Autodesk Inventor part; units mm, degrees
(part 2 of 3)
sketch "Sketch15" plane through (0, 0, 304.8) normal (0, 0, 1) x (1, 0, 0)
  arc A0 (-46.3112, 3289.8328) -> (-107.6796, 3264.8246) centre (12.3811, 3058.0053) ccw
  arc A1 (-107.6796, 3264.8246) -> (-166.2681, 3221.918) centre (64.3962, 2968.4026) ccw
  arc A2 (-166.2681, 3221.918) -> (-212.0324, 3170.0211) centre (46.0659, 2988.5486) ccw
  arc A3 (-212.0324, 3170.0211) -> (-234.7582, 3118.3718) centre (-94.8804, 3087.6496) ccw
  arc A4 (-240.3697, 3101.0693) -> (-234.7582, 3118.3718) centre (-326.0966, 3138.4331) ccw
  arc A5 (-248.2053, 3093.022) -> (-240.3697, 3101.0693) centre (-254.9435, 3107.4212) ccw
  arc A6 (-262.3292, 3089.5785) -> (-248.2053, 3093.022) centre (-263.8246, 3126.4001) ccw
  arc A7 (-297.9256, 3088.8125) -> (-262.3292, 3089.5785) centre (-300.2034, 4022.1257) ccw
  arc A8 (-297.9256, 3088.8125) -> (-398.3817, 3086.3759) centre (-292.3004, 784.8853) ccw
  arc A9 (-398.3817, 3086.3759) -> (-582.9034, 3077.1219) centre (652.3851, -19709.8746) ccw
  arc A10 (-582.9034, 3077.1219) -> (-779.8872, 3065.5252) centre (566.6285, -18127.8528) ccw
  arc A11 (-779.8872, 3065.5252) -> (-944.631, 3053.7542) centre (-115.3773, -7393.4842) ccw
  arc A12 (-944.631, 3053.7542) -> (-1250.7142, 3024.3128) centre (-215.4099, -6133.2828) ccw
  arc A13 (-1250.7142, 3024.3128) -> (-1574.5871, 2983.1171) centre (64.6721, -8610.7314) ccw
  arc A14 (-1574.5871, 2983.1171) -> (-1876.7817, 2935.965) centre (-80.0841, -7586.984) ccw
  arc A15 (-1876.7817, 2935.965) -> (-2112.8509, 2888.5788) centre (-1177.7038, -1158.4352) ccw
  arc A16 (-2163.2488, 2877.2292) -> (-2112.8509, 2888.5788) centre (-3155.0339, 7398.8142) ccw
  arc A17 (-2208.5733, 2867.6541) -> (-2163.2488, 2877.2292) centre (-2805.2472, 5804.1243) ccw
  arc A18 (-2246.7459, 2860.0907) -> (-2208.5733, 2867.6541) centre (-3005.4604, 6789.4539) ccw
  arc A19 (-2258.6611, 2858.9509) -> (-2246.7459, 2860.0907) centre (-2258.6611, 2921.7997) ccw
  arc A20 (-2266.3764, 2860.7683) -> (-2258.6611, 2858.9509) centre (-2258.6611, 2876.2361) ccw
  arc A21 (-2275.0416, 2866.3453) -> (-2266.3764, 2860.7683) centre (-2245.2702, 2903.0826) ccw
  arc A22 (-2283.2654, 2874.4944) -> (-2275.0416, 2866.3453) centre (-2238.4614, 2911.4846) ccw
  arc A23 (-2289.7233, 2884.1233) -> (-2283.2654, 2874.4944) centre (-2238.2095, 2911.6926) ccw
  arc A24 (-2289.7233, 2884.1233) -> (-2321.8745, 2924.2434) centre (-2413.4792, 2817.891) ccw
  arc A25 (-2321.8745, 2924.2434) -> (-2371.8848, 2958.161) centre (-2493.5929, 2724.8793) ccw
  arc A26 (-2371.8848, 2958.161) -> (-2431.0862, 2981.1586) centre (-2505.2634, 2702.5101) ccw
  arc A27 (-2431.0862, 2981.1586) -> (-2490.6497, 2988.9509) centre (-2490.6498, 2757.4058) ccw
  arc A28 (-2490.6497, 2988.9509) -> (-2542.4535, 2985.3232) centre (-2490.6494, 2617.2557) ccw
  arc A29 (-2542.4535, 2985.3232) -> (-2586.7085, 2974.3691) centre (-2511.4982, 2765.3889) ccw
  arc A30 (-2586.7085, 2974.3691) -> (-2626.6985, 2954.9638) centre (-2515.7885, 2777.3109) ccw
  arc A31 (-2626.6985, 2954.9638) -> (-2665.6409, 2925.9729) centre (-2469.4507, 2703.0889) ccw
  arc A32 (-2665.6409, 2925.9729) -> (-2702.3557, 2887.9704) centre (-2449.4743, 2680.3944) ccw
  arc A33 (-2702.3557, 2887.9704) -> (-2729.3602, 2847.2341) centre (-2516.7134, 2735.5871) ccw
  arc A34 (-2729.3602, 2847.2341) -> (-2747.2851, 2802.3677) centre (-2522.1108, 2738.4208) ccw
  arc A35 (-2747.2851, 2802.3677) -> (-2756.9469, 2752.0682) centre (-2463.5322, 2721.785) ccw
  line L0 (-2756.9469, 2752.0682) -> (-2762.5543, 2697.7376)
  line L1 (-2762.5543, 2697.7376) -> (-2857.3018, 2653.4618)
  arc A36 (-2857.3018, 2653.4618) -> (-2992.0543, 2581.5731) centre (-2246.1893, 1345.7176) ccw
  arc A37 (-2992.0543, 2581.5731) -> (-3103.2533, 2502.66) centre (-2516.6696, 1793.8896) ccw
  arc A38 (-3103.2533, 2502.66) -> (-3188.8522, 2418.6621) centre (-2650.8401, 1956.0099) ccw
  arc A39 (-3188.8522, 2418.6621) -> (-3246.4159, 2331.4275) centre (-2875.8904, 2149.5375) ccw
  line L2 (-3246.4159, 2331.4275) -> (-3274.631, 2273.9509)
  line L3 (-3274.631, 2273.9509) -> (-3274.631, 1968.9509)
  arc A40 (-3274.631, 1968.9509) -> (-3273.1115, 1744.3083) centre (13331.6928, 1968.9509) ccw
  arc A41 (-3273.1115, 1744.3083) -> (-3264.9339, 1658.0418) centre (-2737.5712, 1751.554) ccw
  arc A42 (-3264.9339, 1658.0418) -> (-3243.4484, 1598.0315) centre (-3077.6061, 1691.2592) ccw
  arc A43 (-3243.4484, 1598.0315) -> (-3196.1509, 1526.3644) centre (-2717.5396, 1893.6705) ccw
  line L4 (-3196.1509, 1526.3644) -> (-3159.631, 1478.7779)
  line L5 (-3159.631, 1478.7779) -> (-3159.631, 232.7481)
  line L6 (-3159.631, 232.7481) -> (-3159.631, -1013.2817)
  line L7 (-3159.631, -1013.2817) -> (-3194.6687, -1106.8292)
  arc A44 (-3194.6687, -1106.8292) -> (-3235.7053, -1228.3112) centre (-1352.9181, -1796.6438) ccw
  arc A45 (-3235.7053, -1228.3112) -> (-3254.4602, -1317.8486) centre (-2729.893, -1380.9943) ccw
  arc A46 (-3254.4602, -1317.8486) -> (-3262.6146, -1433.5138) centre (-2089.2145, -1458.1182) ccw
  arc A47 (-3262.6146, -1433.5138) -> (-3266.9659, -1707.4159) centre (23693.9, -1998.7406) ccw
  arc A48 (-3266.9659, -1707.4159) -> (-3268.5559, -1915.4498) centre (29628.1072, -2062.8585) ccw
  arc A49 (-3268.5559, -1915.4498) -> (-3267.3161, -2035.0331) centre (758.7581, -1933.4937) ccw
  arc A50 (-3267.3161, -2035.0331) -> (-3263.1758, -2116.2659) centre (-1685.718, -1995.1434) ccw
  arc A51 (-3263.1758, -2116.2659) -> (-3254.9956, -2182.0248) centre (-2561.9283, -2062.4215) ccw
  arc A52 (-3254.9956, -2182.0248) -> (-3203.1859, -2382.1563) centre (-2017.8834, -1968.535) ccw
  arc A53 (-3203.1859, -2382.1563) -> (-3118.1576, -2576.8834) centre (-1881.2535, -1920.8569) ccw
  arc A54 (-3118.1576, -2576.8834) -> (-3000.6889, -2764.0458) centre (-1776.8359, -1865.4747) ccw
  arc A55 (-3000.6889, -2764.0458) -> (-2852.131, -2941.6043) centre (-1527.6023, -1682.4847) ccw
  line L8 (-2852.131, -2941.6043) -> (-2759.631, -3038.9096)
  line L9 (-2759.631, -3038.9096) -> (-2759.631, -3148.0159)
  arc A56 (-2759.631, -3148.0159) -> (-2758.7481, -3211.3797) centre (-485.5874, -3148.0178) ccw
  arc A57 (-2758.7481, -3211.3797) -> (-2755.3551, -3247.6045) centre (-2481.0428, -3203.6394) ccw
  arc A58 (-2755.3551, -3247.6045) -> (-2747.9013, -3276.2194) centre (-2602.9015, -3223.1703) ccw
  arc A59 (-2747.9013, -3276.2194) -> (-2733.8535, -3308.8509) centre (-2448.718, -3166.7618) ccw
  arc A60 (-2733.8535, -3308.8509) -> (-2656.0182, -3402.6512) centre (-2494.9406, -3189.7953) ccw
  arc A61 (-2656.0182, -3402.6512) -> (-2544.9951, -3451.4517) centre (-2497.9927, -3193.8282) ccw
  arc A62 (-2544.9951, -3451.4517) -> (-2424.0985, -3444.948) centre (-2498.1767, -3194.8371) ccw
  arc A63 (-2424.0985, -3444.948) -> (-2318.7115, -3384.5922) centre (-2499.0501, -3191.8895) ccw
  line L10 (-2318.7115, -3384.5922) -> (-2292.792, -3360.3356)
  line L11 (-2292.792, -3360.3356) -> (-2228.7115, -3394.9426)
  arc A64 (-2228.7115, -3394.9426) -> (-2141.5432, -3438.4245) centre (-1515.7339, -2074.7467) ccw
  arc A65 (-2141.5432, -3438.4245) -> (-2023.9363, -3490.359) centre (-279.2994, 619.5343) ccw
  arc A66 (-2023.9363, -3490.359) -> (-1897.8735, -3541.7652) centre (-157.0169, 907.5921) ccw
  arc A67 (-1897.8735, -3541.7652) -> (-1782.4495, -3584.3792) centre (-735.1306, -569.9907) ccw
  arc A68 (-1782.4495, -3584.3792) -> (-1501.5658, -3670.687) centre (-452.9966, 242.0338) ccw
  arc A69 (-1501.5658, -3670.687) -> (-1204.3636, -3740.1039) centre (-281.5333, 881.8376) ccw
  arc A70 (-1204.3636, -3740.1039) -> (-893.0578, -3792.182) centre (-217.5273, 1202.3994) ccw
  arc A71 (-893.0578, -3792.182) -> (-569.8728, -3826.4861) centre (-133.7905, 1821.478) ccw
  arc A72 (-319.0343, -3846.0577) -> (-569.8728, -3826.4861) centre (-12555.6397, -159058.0844) ccw
  arc A73 (-268.9912, -3851.9794) -> (-319.0343, -3846.0577) centre (-369.6818, -4488.4814) ccw
  arc A74 (-247.4204, -3861.4112) -> (-268.9912, -3851.9794) centre (-276.2744, -3898.0189) ccw
  arc A75 (-236.4852, -3879.2256) -> (-247.4204, -3861.4112) centre (-266.1467, -3885.1696) ccw
  arc A76 (-236.4852, -3879.2256) -> (-224.011, -3912.1165) centre (-131.3204, -3858.1516) ccw
  arc A77 (-224.011, -3912.1165) -> (-197.1839, -3951.7522) centre (81.3306, -3734.3454) ccw
  arc A78 (-197.1839, -3951.7522) -> (-163.6615, -3989.2021) centre (97.3029, -3721.8771) ccw
  arc A79 (-163.6615, -3989.2021) -> (-129.7306, -4015.9862) centre (-19.7812, -3841.8149) ccw
  arc A80 (-129.7306, -4015.9862) -> (-22.8543, -4054.6276) centre (11.689, -3791.9632) ccw
  arc A81 (-22.8543, -4054.6276) -> (89.6103, -4044.5426) centre (10.8492, -3798.3496) ccw
  arc A82 (89.6103, -4044.5426) -> (188.2078, -3987.1875) centre (8.9809, -3792.5094) ccw
  arc A83 (188.2078, -3987.1875) -> (255.8747, -3892.625) centre (-4.6846, -3777.6663) ccw
  arc A84 (274.2339, -3865.5547) -> (255.8747, -3892.625) centre (339.2509, -3929.4105) ccw
  arc A85 (298.361, -3852.3578) -> (274.2339, -3865.5547) centre (308.0992, -3898.8151) ccw
  arc A86 (346.2469, -3845.5982) -> (298.361, -3852.3578) centre (373.1383, -4209.0913) ccw
  arc A87 (550.369, -3830.8943) -> (346.2469, -3845.5982) centre (4245.7889, -56555.6607) ccw
  arc A88 (550.369, -3830.8943) -> (1011.9622, -3779.143) centre (160.6183, 1729.9233) ccw
  arc A89 (1011.9622, -3779.143) -> (1450.7614, -3690.264) centre (276.8483, 977.7708) ccw
  arc A90 (1450.7614, -3690.264) -> (1856.9933, -3566.6691) centre (393.1521, 515.2843) ccw
  arc A91 (1856.9933, -3566.6691) -> (2220.8715, -3410.7969) centre (749.9478, -479.643) ccw
  line L12 (2220.8715, -3410.7969) -> (2317.8832, -3362.1141)
  line L13 (2317.8832, -3362.1141) -> (2340.395, -3386.0768)
  arc A92 (2340.395, -3386.0768) -> (2398.6598, -3427.8945) centre (2475.8998, -3258.7765) ccw
  arc A93 (2398.6598, -3427.8945) -> (2476.161, -3451.1721) centre (2522.0514, -3157.7269) ccw
  arc A94 (2476.161, -3451.1721) -> (2558.9087, -3452.9409) centre (2524.1075, -3144.5807) ccw
  arc A95 (2558.9087, -3452.9409) -> (2632.5758, -3431.7696) centre (2533.124, -3224.4709) ccw
  arc A96 (2632.5758, -3431.7696) -> (2672.6678, -3407.2012) centre (2533.1516, -3224.5277) ccw
  arc A97 (2672.6678, -3407.2012) -> (2711.9464, -3372.3297) centre (2456.4615, -3124.1138) ccw
  arc A98 (2711.9464, -3372.3297) -> (2745.4004, -3332.3528) centre (2459.6723, -3127.2323) ccw
  arc A99 (2745.4004, -3332.3528) -> (2767.9369, -3292.4447) centre (2573.5904, -3209.0123) ccw
  arc A100 (2767.9369, -3292.4447) -> (2774.851, -3270.202) centre (2664.9715, -3248.2421) ccw
  arc A101 (2774.851, -3270.202) -> (2780.6818, -3235.3215) centre (2226.4162, -3160.5947) ccw
  arc A102 (2780.6818, -3235.3215) -> (2785.2966, -3191.8844) centre (2012.2156, -3131.7156) ccw
  arc A103 (2785.2966, -3191.8844) -> (2788.3077, -3141.3505) centre (1395.4115, -3083.711) ccw
  line L14 (2788.3077, -3141.3505) -> (2793.054, -3026.652)
  line L15 (2793.054, -3026.652) -> (2881.9987, -2931.3505)
  arc A104 (2881.9987, -2931.3505) -> (3026.1461, -2756.7165) centre (1521.0591, -1661.188) ccw
  arc A105 (3026.1461, -2756.7165) -> (3141.0373, -2573.2817) centre (1768.6588, -1841.4137) ccw
  arc A106 (3141.0373, -2573.2817) -> (3224.9271, -2383.8991) centre (1886.8926, -1904.4681) ccw
  arc A107 (3224.9271, -2383.8991) -> (3276.549, -2191.4998) centre (2079.1422, -1973.3533) ccw
  arc A108 (3276.549, -2191.4998) -> (3290.3678, -2067.3509) centre (2389.8588, -2029.96) ccw
  arc A109 (3290.3678, -2067.3509) -> (3297.8944, -1821.3895) centre (-7979.8895, -1599.3782) ccw
  arc A110 (3297.8944, -1821.3895) -> (3299.7736, -1574.0698) centre (-6932.4546, -1619.9901) ccw
  arc A111 (3299.7736, -1574.0698) -> (3291.643, -1424.7762) centre (1801.6108, -1580.7922) ccw
  arc A112 (3291.643, -1424.7762) -> (3279.1795, -1335.9693) centre (2021.1062, -1557.8098) ccw
  arc A113 (3279.1795, -1335.9693) -> (3260.4248, -1247.3936) centre (1972.1003, -1566.4515) ccw
  arc A114 (3260.4248, -1247.3936) -> (3235.7287, -1160.5183) centre (1978.3425, -1564.905) ccw
  arc A115 (3235.7287, -1160.5183) -> (3205.467, -1076.8057) centre (2049.2486, -1542.0999) ccw
  line L16 (3205.467, -1076.8057) -> (3177.6016, -1007.5624)
  line L17 (3177.6016, -1007.5624) -> (3183.3958, 240.5471)
  line L18 (3183.3958, 240.5471) -> (3189.19, 1488.6566)
  line L19 (3189.19, 1488.6566) -> (3220.1008, 1527.121)
  arc A116 (3220.1008, 1527.121) -> (3233.5209, 1545.7307) centre (3048.6242, 1664.9232) ccw
  arc A117 (3233.5209, 1545.7307) -> (3248.3718, 1570.2027) centre (2790.547, 1831.2912) ccw
  arc A118 (3248.3718, 1570.2027) -> (3262.2919, 1596.2159) centre (2772.5487, 1841.5547) ccw
  arc A119 (3262.2919, 1596.2159) -> (3272.9357, 1619.7682) centre (2973.0626, 1741.1062) ccw
  arc A120 (3272.9357, 1619.7682) -> (3285.3139, 1660.1743) centre (3048.0912, 1710.7471) ccw
  arc A121 (3285.3139, 1660.1743) -> (3292.0528, 1706.3262) centre (2934.4481, 1734.9744) ccw
  arc A122 (3292.0528, 1706.3262) -> (3295.7316, 1779.1786) centre (2058.9549, 1805.1132) ccw
  arc A123 (3295.7316, 1779.1786) -> (3298.506, 1938.9509) centre (-18868.7762, 2243.9706) ccw
  arc A124 (3298.506, 1938.9509) -> (3299.3295, 2124.9239) centre (-6667.2613, 2076.0683) ccw
  arc A125 (3299.3295, 2124.9239) -> (3293.7335, 2225.5886) centre (2303.2827, 2120.0404) ccw
  arc A126 (3293.7335, 2225.5886) -> (3279.7247, 2296.0862) centre (2896.0955, 2183.2137) ccw
  arc A127 (3279.7247, 2296.0862) -> (3253.3427, 2362.7578) centre (2899.7829, 2184.2986) ccw
  arc A128 (3253.3427, 2362.7578) -> (3201.8504, 2436.6131) centre (2968.2007, 2218.8331) ccw
  arc A129 (3201.8504, 2436.6131) -> (3120.5863, 2511.187) centre (2684.435, 1954.3428) ccw
  arc A130 (3120.5863, 2511.187) -> (3012.8103, 2584.6184) centre (2514.227, 1737.0353) ccw
  arc A131 (3012.8103, 2584.6184) -> (2880.2295, 2655.0014) centre (2141.5699, 1103.522) ccw
  line L20 (2880.2295, 2655.0014) -> (2780.369, 2702.545)
  line L21 (2780.369, 2702.545) -> (2780.1493, 2748.2479)
  arc A132 (2780.1493, 2748.2479) -> (2775.0931, 2791.6815) centre (2582.9337, 2747.3004) ccw
  arc A133 (2775.0931, 2791.6815) -> (2760.5416, 2834.592) centre (2553.9, 2740.5949) ccw
  arc A134 (2760.5416, 2834.592) -> (2737.1518, 2875.1119) centre (2539.7972, 2734.1798) ccw
  arc A135 (2737.1518, 2875.1119) -> (2705.9098, 2911.4545) centre (2520.0411, 2720.0719) ccw
  arc A136 (2705.9098, 2911.4545) -> (2667.4339, 2943.5189) centre (2476.1982, 2674.9279) ccw
  arc A137 (2667.4339, 2943.5189) -> (2628.0644, 2965.8563) centre (2539.3212, 2763.5843) ccw
  arc A138 (2628.0644, 2965.8563) -> (2584.5734, 2979.8878) centre (2537.3397, 2759.0682) ccw
  arc A139 (2584.5734, 2979.8878) -> (2533.6971, 2987.0098) centre (2509.5141, 2628.9801) ccw
  arc A140 (2533.6971, 2987.0098) -> (2468.8699, 2982.8618) centre (2516.9837, 2739.5663) ccw
  arc A141 (2468.8699, 2982.8618) -> (2406.3831, 2962.0597) centre (2519.6551, 2726.0573) ccw
  arc A142 (2406.3831, 2962.0597) -> (2350.9834, 2926.2821) centre (2519.9793, 2725.382) ccw
  arc A143 (2350.9834, 2926.2821) -> (2306.9568, 2878.1833) centre (2512.6195, 2734.1315) ccw
  line L22 (2306.9568, 2878.1833) -> (2291.8513, 2856.6172)
  line L23 (2291.8513, 2856.6172) -> (2153.3688, 2887.2409)
  arc A144 (2153.3688, 2887.2409) -> (1789.0499, 2956.0222) centre (863.5291, -2945.494) ccw
  arc A145 (1789.0499, 2956.0222) -> (1366.7853, 3013.4039) centre (178.3761, -7314.3462) ccw
  arc A146 (1366.7853, 3013.4039) -> (909.4742, 3057.1147) centre (4.1851, -8828.2906) ccw
  arc A147 (909.4742, 3057.1147) -> (438.4615, 3084.5728) centre (-97.6129, -10164.7522) ccw
  line L24 (438.4615, 3084.5728) -> (271.5539, 3091.326)
  line L25 (271.5539, 3091.326) -> (245.4506, 3144.6794)
  arc A148 (245.4506, 3144.6794) -> (194.1184, 3215.755) centre (13.3359, 3031.1162) ccw
  arc A149 (194.1184, 3215.755) -> (120.5657, 3268.0706) centre (-8.3291, 3008.9888) ccw
  arc A150 (120.5657, 3268.0706) -> (36.2378, 3294.2646) centre (-2.5085, 3020.6882) ccw
  arc A151 (36.2378, 3294.2646) -> (-46.3112, 3289.8328) centre (6.2222, 3082.3333) ccw
  arc A152 (89.3189, 3150.4436) -> (63.1902, 3165.2397) centre (10.7465, 3042.1598) ccw
  arc A153 (116.9335, 3127.4656) -> (89.3189, 3150.4436) centre (-69.9138, 2930.998) ccw
  arc A154 (138.8775, 3104.1724) -> (116.9335, 3127.4656) centre (-83.9919, 2916.1953) ccw
  arc A155 (138.4328, 3093.6815) -> (138.8775, 3104.1724) centre (132.9453, 3099.1689) ccw
  arc A156 (133.5538, 3091.581) -> (138.4328, 3093.6815) centre (133.3552, 3098.7591) ccw
  arc A157 (97.1027, 3090.7293) -> (133.5538, 3091.581) centre (16.2051, 7333.5774) ccw
  arc A158 (54.6327, 3090.4516) -> (97.1027, 3090.7293) centre (64.784, 4785.7998) ccw
  arc A159 (5.2451, 3091.142) -> (54.6327, 3090.4516) centre (73.1416, 6181.3364) ccw
  line L26 (5.2451, 3091.142) -> (-122.5944, 3093.9509)
  line L27 (-122.5944, 3093.9509) -> (-95.2836, 3126.3799)
  arc A160 (-61.8221, 3155.7464) -> (-95.2836, 3126.3799) centre (18.2392, 3030.774) ccw
  arc A161 (-22.1385, 3172.7641) -> (-61.8221, 3155.7464) centre (9.2314, 3044.835) ccw
  arc A162 (20.6657, 3175.9635) -> (-22.1385, 3172.7641) centre (8.8195, 3046.5143) ccw
  arc A163 (63.1902, 3165.2397) -> (20.6657, 3175.9635) centre (7.7851, 3035.21) ccw
  arc A164 (1482.1495, 2879.5394) -> (835.369, 2944.786) centre (-222.8049, -10783.103) ccw
  arc A165 (2033.8348, 2789.8546) -> (1482.1495, 2879.5394) centre (546.8422, -4615.54) ccw
  arc A166 (2488.7788, 2677.7909) -> (2033.8348, 2789.8546) centre (969.6677, -2509.8371) ccw
  arc A167 (2835.369, 2543.1909) -> (2488.7788, 2677.7909) centre (1877.3908, 589.9613) ccw
  arc A168 (2972.4358, 2468.9016) -> (2835.369, 2543.1909) centre (1991.5457, 822.7108) ccw
  arc A169 (3070.8462, 2398.2555) -> (2972.4358, 2468.9016) centre (2608.3198, 1857.8197) ccw
  arc A170 (3136.2171, 2328.1438) -> (3070.8462, 2398.2555) centre (2793.243, 2073.8919) ccw
  arc A171 (3171.2321, 2255.7454) -> (3136.2171, 2328.1438) centre (2962.8708, 2199.6394) ccw
  arc A172 (3167.3401, 2165.8281) -> (3171.2321, 2255.7454) centre (3027.1211, 2216.9403) ccw
  arc A173 (3112.4013, 2072.38) -> (3167.3401, 2165.8281) centre (2885.8896, 2268.4214) ccw
  arc A174 (3006.3187, 1977.6944) -> (3112.4013, 2072.38) centre (2693.5168, 2434.916) ccw
  arc A175 (2849.8778, 1884.4435) -> (3006.3187, 1977.6944) centre (2182.6997, 3181.5742) ccw
  line L28 (2849.8778, 1884.4435) -> (2744.3866, 1830.1842)
  line L29 (2744.3866, 1830.1842) -> (2718.8658, 1862.1684)
  arc A176 (2718.8658, 1862.1684) -> (2705.319, 1876.4972) centre (2626.883, 1788.7735) ccw
  arc A177 (2705.319, 1876.4972) -> (2685.042, 1893.3565) centre (2460.6821, 1602.8924) ccw
  arc A178 (2685.042, 1893.3565) -> (2662.0222, 1909.8756) centre (2439.3453, 1575.269) ccw
  arc A179 (2662.0222, 1909.8756) -> (2639.5587, 1923.4268) centre (2498.2071, 1663.7176) ccw
  arc A180 (2639.5587, 1923.4268) -> (2522.8271, 1952.9332) centre (2523.618, 1710.4053) ccw
  arc A181 (2522.8271, 1952.9332) -> (2402.6794, 1924.0014) centre (2523.6996, 1685.3691) ccw
  arc A182 (2402.6794, 1924.0014) -> (2308.0062, 1844.0185) centre (2524.5087, 1683.7737) ccw
  arc A183 (2308.0062, 1844.0185) -> (2261.9871, 1731.9451) centre (2506.7243, 1696.9371) ccw
  line L30 (2261.9871, 1731.9451) -> (2255.1849, 1684.392)
  line L31 (2255.1849, 1684.392) -> (2180.277, 1666.9309)
  arc A184 (2080.1328, 1646.3683) -> (2180.277, 1666.9309) centre (1742.2701, 3545.9722) ccw
  arc A185 (1895.2662, 1614.4296) -> (2080.1328, 1646.3683) centre (-1243.6324, 20333.9108) ccw
  arc A186 (1705.5784, 1583.7089) -> (1895.2662, 1614.4296) centre (-954.2792, 18608.2412) ccw
  arc A187 (1570.369, 1564.661) -> (1705.5784, 1583.7089) centre (1004.2625, 6072.516) ccw
  arc A188 (1325.9578, 1537.6216) -> (1570.369, 1564.661) centre (531.3741, 9838.0633) ccw
  arc A189 (1053.4411, 1514.482) -> (1325.9578, 1537.6216) centre (111.4621, 14224.5078) ccw
  arc A190 (765.7527, 1496.1277) -> (1053.4411, 1514.482) centre (15.6875, 15516.6442) ccw
  arc A191 (475.369, 1483.5075) -> (765.7527, 1496.1277) centre (-9.5547, 15988.3407) ccw
  line L32 (475.369, 1483.5075) -> (275.369, 1476.8212)
  line L33 (275.369, 1476.8212) -> (254.0585, 1520.7051)
  arc A192 (254.0585, 1520.7051) -> (210.3619, 1589.1404) centre (-60.9732, 1367.7223) ccw
  arc A193 (210.3619, 1589.1404) -> (155.3377, 1638.8441) centre (20.3039, 1434.0467) ccw
  arc A194 (155.3377, 1638.8441) -> (89.5075, 1668.7278) centre (27.9039, 1445.5724) ccw
  arc A195 (89.5075, 1668.7278) -> (14.0565, 1678.9509) centre (14.0566, 1395.4107) ccw
  arc A196 (14.0565, 1678.9509) -> (-11.8929, 1678.1751) centre (14.0563, 1244.6069) ccw
  arc A197 (-11.8929, 1678.1751) -> (-38.2726, 1675.8493) centre (16.1999, 1208.7817) ccw
  arc A198 (-38.2726, 1675.8493) -> (-61.5157, 1672.4671) centre (9.6394, 1265.031) ccw
  arc A199 (-61.5157, 1672.4671) -> (-76.48, 1668.3921) centre (-47.1455, 1590.1833) ccw
  arc A200 (-76.48, 1668.3921) -> (-128.8275, 1641.0381) centre (8.2697, 1442.4402) ccw
  arc A201 (-128.8275, 1641.0381) -> (-177.1616, 1600.019) centre (52.4265, 1378.4747) ccw
  arc A202 (-177.1616, 1600.019) -> (-214.9194, 1551.8877) centre (38.2305, 1392.1732) ccw
  arc A203 (-214.9194, 1551.8877) -> (-235.6528, 1503.44) centre (-73.7028, 1462.793) ccw
  line L34 (-235.6528, 1503.44) -> (-242.4619, 1476.3107)
  line L35 (-242.4619, 1476.3107) -> (-443.5464, 1482.9751)
  arc A204 (-781.6776, 1498.1041) -> (-443.5464, 1482.9751) centre (40.3784, 16084.7975) ccw
  arc A205 (-1113.5104, 1520.8708) -> (-781.6776, 1498.1041) centre (-15.0259, 15102.0022) ccw
  arc A206 (-1424.5661, 1550.0611) -> (-1113.5104, 1520.8708) centre (-134.3343, 13627.0071) ccw
  arc A207 (-1699.631, 1584.5707) -> (-1424.5661, 1550.0611) centre (-623.2941, 9050.2236) ccw
  arc A208 (-1847.5677, 1607.9222) -> (-1699.631, 1584.5707) centre (-900.4908, 7127.5823) ccw
  arc A209 (-2024.8783, 1639.7582) -> (-1847.5677, 1607.9222) centre (122.9979, 13092.6605) ccw
  arc A210 (-2203.0789, 1673.6057) -> (-2024.8783, 1639.7582) centre (5187.0232, 40095.073) ccw
  arc A211 (-2229.6676, 1683.9735) -> (-2203.0789, 1673.6057) centre (-2188.1699, 1751.1182) ccw
  arc A212 (-2233.5296, 1688.4289) -> (-2229.6676, 1683.9735) centre (-2224.4739, 1692.3771) ccw
  arc A213 (-2236.7688, 1697.696) -> (-2233.5296, 1688.4289) centre (-2173.3861, 1714.6508) ccw
  arc A214 (-2239.0342, 1709.3739) -> (-2236.7688, 1697.696) centre (-2154.3459, 1719.7441) ccw
  arc A215 (-2239.8507, 1722.0411) -> (-2239.0342, 1709.3739) centre (-2129.3798, 1722.8013) ccw
  arc A216 (-2239.8507, 1722.0411) -> (-2241.3449, 1737.4255) centre (-2325.8938, 1721.4489) ccw
  arc A217 (-2241.3449, 1737.4255) -> (-2245.9894, 1757.7962) centre (-2515.8192, 1685.5599) ccw
  arc A218 (-2245.9894, 1757.7962) -> (-2252.6251, 1779.3829) centre (-2543.6586, 1678.1075) ccw
  arc A219 (-2252.6251, 1779.3829) -> (-2260.4402, 1798.9509) centre (-2473.353, 1702.5729) ccw
  arc A220 (-2260.4402, 1798.9509) -> (-2321.3408, 1884.0844) centre (-2505.4017, 1688.0659) ccw
  arc A221 (-2321.3408, 1884.0844) -> (-2409.2894, 1937.9452) centre (-2495.1954, 1698.9352) ccw
  arc A222 (-2409.2894, 1937.9452) -> (-2511.3892, 1952.3913) centre (-2495.1682, 1699.0108) ccw
  arc A223 (-2511.3892, 1952.3913) -> (-2612.5139, 1925.4945) centre (-2494.228, 1684.3206) ccw
  arc A224 (-2612.5139, 1925.4945) -> (-2636.2509, 1912.4906) centre (-2480.6136, 1656.5615) ccw
  arc A225 (-2636.2509, 1912.4906) -> (-2659.7087, 1896.9032) centre (-2453.818, 1612.4982) ccw
  arc A226 (-2659.7087, 1896.9032) -> (-2679.6838, 1881.1529) centre (-2478.0925, 1646.0292) ccw
  arc A227 (-2679.6838, 1881.1529) -> (-2691.8945, 1868.0281) centre (-2627.8055, 1820.645) ccw
  arc A228 (-2701.1026, 1856.898) -> (-2691.8945, 1868.0281) centre (-2798.4403, 1946.8009) ccw
  arc A229 (-2710.9898, 1847.4924) -> (-2701.1026, 1856.898) centre (-2778.7017, 1928.5703) ccw
  arc A230 (-2720.1773, 1840.8276) -> (-2710.9898, 1847.4924) centre (-2764.3515, 1911.3875) ccw
  arc A231 (-2726.7114, 1838.9509) -> (-2720.1773, 1840.8276) centre (-2726.7114, 1851.2646) ccw
  arc A232 (-2753.7237, 1845.3018) -> (-2726.7114, 1838.9509) centre (-2726.7114, 1899.5727) ccw
  arc A233 (-2840.5324, 1889.6133) -> (-2753.7237, 1845.3018) centre (-613.0566, 6146.167) ccw
  arc A234 (-2925.9549, 1936.3835) -> (-2840.5324, 1889.6133) centre (-1640.6562, 4182.5004) ccw
  arc A235 (-2985.1408, 1974.188) -> (-2925.9549, 1936.3835) centre (-2567.4658, 2562.8588) ccw
  arc A236 (-3082.6143, 2057.1523) -> (-2985.1408, 1974.188) centre (-2564.0881, 2567.6185) ccw
  arc A237 (-3138.0866, 2139.3854) -> (-3082.6143, 2057.1523) centre (-2889.5513, 2247.2141) ccw
  arc A238 (-3151.8847, 2220.6906) -> (-3138.0866, 2139.3854) centre (-2979.7531, 2208.0793) ccw
  arc A239 (-3126.9127, 2300.9598) -> (-3151.8847, 2220.6906) centre (-2966.8061, 2207.1309) ccw
  arc A240 (-2956.3381, 2468.7845) -> (-3126.9127, 2300.9598) centre (-2730.4953, 2068.6441) ccw
  arc A241 (-2626.8929, 2620.4784) -> (-2956.3381, 2468.7845) centre (-1872.4141, 548.3318) ccw
  arc A242 (-2171.9284, 2752.7897) -> (-2626.8929, 2620.4784) centre (-1401.1451, -745.9926) ccw
  arc A243 (-1595.2352, 2858.6522) -> (-2171.9284, 2752.7897) centre (-384.2402, -5362.0464) ccw
  arc A244 (-1392.8844, 2885.7315) -> (-1595.2352, 2858.6522) centre (-470.2354, -4778.3656) ccw
  arc A245 (-1159.536, 2911.7617) -> (-1392.8844, 2885.7315) centre (217.0043, -10487.205) ccw
  arc A246 (-925.1701, 2933.7788) -> (-1159.536, 2911.7617) centre (222.1026, -10536.9988) ccw
  arc A247 (-719.631, 2948.6064) -> (-925.1701, 2933.7788) centre (-249.8427, -4995.572) ccw
  arc A248 (-719.631, 2948.6064) -> (-645.1354, 2953.0514) centre (-4891.6254, 73495.9092) ccw
  arc A249 (-645.1354, 2953.0514) -> (-574.2873, 2957.3599) centre (-4118.3267, 60649.1253) ccw
  arc A250 (-574.2873, 2957.3599) -> (-514.3278, 2961.0761) centre (-3947.3842, 57867.181) ccw
  arc A251 (-514.3278, 2961.0761) -> (-484.631, 2963.0426) centre (-766.6687, 6996.9302) ccw
  arc A252 (-310.3321, 2968.445) -> (-484.631, 2963.0426) centre (-327.9324, 721.8583) ccw
  arc A253 (157.5377, 2963.377) -> (-310.3321, 2968.445) centre (-921.6305, -75064.2439) ccw
  arc A254 (620.3058, 2955.3224) -> (157.5377, 2963.377) centre (-737.9031, -61781.3585) ccw
  arc A255 (835.369, 2944.786) -> (620.3058, 2955.3224) centre (539.5761, -892.6274) ccw
  line L36 (-2415.4337, 2843.5667) -> (-2386.2364, 2824.4265)
  line L37 (-2386.2364, 2824.4265) -> (-2508.906, 2785.9943)
  arc A256 (-2556.3683, 2771.7015) -> (-2508.906, 2785.9943) centre (-3175.859, 4914.8005) ccw
  arc A257 (-2597.3301, 2760.6403) -> (-2556.3683, 2771.7015) centre (-2890.2085, 3926.6021) ccw
  arc A258 (-2632.2704, 2752.1202) -> (-2597.3301, 2760.6403) centre (-3230.5872, 5281.6688) ccw
  arc A259 (-2637.6648, 2753.6513) -> (-2632.2704, 2752.1202) centre (-2633.5952, 2757.7209) ccw
  arc A260 (-2639.9242, 2767.33) -> (-2637.6648, 2753.6513) centre (-2629.2487, 2762.0674) ccw
  arc A261 (-2621.792, 2799.3086) -> (-2639.9242, 2767.33) centre (-2354.5921, 2626.6733) ccw
  arc A262 (-2597.9264, 2831.1582) -> (-2621.792, 2799.3086) centre (-2380.9161, 2643.6815) ccw
  arc A263 (-2574.6718, 2851.1502) -> (-2597.9264, 2831.1582) centre (-2519.3379, 2763.2652) ccw
  arc A264 (-2541.0487, 2863.9713) -> (-2574.6718, 2851.1502) centre (-2525.8434, 2773.5978) ccw
  arc A265 (-2496.6675, 2866.6174) -> (-2541.0487, 2863.9713) centre (-2506.5565, 2658.9647) ccw
  arc A266 (-2451.5324, 2859.6581) -> (-2496.6675, 2866.6174) centre (-2506.9927, 2649.8104) ccw
  arc A267 (-2415.4337, 2843.5667) -> (-2451.5324, 2859.6581) centre (-2483.042, 2740.4339) ccw
  arc A268 (2620.5832, 2829.9518) -> (2597.9981, 2848.982) centre (2547.4463, 2766.07) ccw
  arc A269 (2643.9164, 2799.1346) -> (2620.5832, 2829.9518) centre (2412.1447, 2647.8903) ccw
  arc A270 (2661.6773, 2768.0955) -> (2643.9164, 2799.1346) centre (2387.5231, 2631.8231) ccw
  arc A271 (2659.4944, 2754.743) -> (2661.6773, 2768.0955) centre (2651.3001, 2762.9373) ccw
  arc A272 (2650.0334, 2752.3821) -> (2659.4944, 2754.743) centre (2652.7984, 2761.439) ccw
  arc A273 (2537.8137, 2786.898) -> (2650.0334, 2752.3821) centre (10875.0686, 29693.7231) ccw
  arc A274 (2425.4147, 2821.9639) -> (2537.8137, 2786.898) centre (11547.2443, 31863.0982) ccw
  arc A275 (2420.369, 2828.8375) -> (2425.4147, 2821.9639) centre (2427.5737, 2828.8375) ccw
  arc A276 (2421.6582, 2831.7939) -> (2420.369, 2828.8375) centre (2424.4034, 2828.8375) ccw
  arc A277 (2428.4471, 2837.717) -> (2421.6582, 2831.7939) centre (2520.607, 2725.2335) ccw
  arc A278 (2437.3333, 2844.4381) -> (2428.4471, 2837.717) centre (2519.3452, 2726.7729) ccw
  arc A279 (2447.869, 2851.3687) -> (2437.3333, 2844.4381) centre (2571.6099, 2651.7874) ccw
  arc A280 (2480.5541, 2864.357) -> (2447.869, 2851.3687) centre (2500.5694, 2766.3684) ccw
  arc A281 (2521.9294, 2868.2076) -> (2480.5541, 2864.357) centre (2518.8849, 2676.7014) ccw
  arc A282 (2563.7901, 2863.0137) -> (2521.9294, 2868.2076) centre (2518.8063, 2671.7481) ccw
  arc A283 (2597.9981, 2848.982) -> (2563.7901, 2863.0137) centre (2536.9354, 2748.8309) ccw
  arc A284 (-3039.5487, 1861.5653) -> (-2992.9976, 1833.2356) centre (-2696.508, 2372.8342) ccw
  arc A285 (-2992.9976, 1833.2356) -> (-2914.1341, 1791.0183) centre (-1022.0162, 5420.3446) ccw
  arc A286 (-2914.1341, 1791.0183) -> (-2834.5715, 1750.6173) centre (-988.9724, 5483.7302) ccw
  arc A287 (-2834.5715, 1750.6173) -> (-2786.6467, 1729.7173) centre (-2592.6718, 2239.9097) ccw
  line L38 (-2786.6467, 1729.7173) -> (-2759.631, 1719.446)
  line L39 (-2759.631, 1719.446) -> (-2759.631, 1534.1984)
  arc A288 (-2760.1701, 1463.1667) -> (-2759.631, 1534.1984) centre (-7440.3636, 1534.2013) ccw
  arc A289 (-2761.8342, 1403.3695) -> (-2760.1701, 1463.1667) centre (-5125.5545, 1499.071) ccw
  arc A290 (-2764.0849, 1351.862) -> (-2761.8342, 1403.3695) centre (-10805.9589, 1729.0655) ccw
  arc A291 (-2767.131, 1348.9582) -> (-2764.0849, 1351.862) centre (-2767.1281, 1352.0048) ccw
  arc A292 (-2784.1053, 1353.6893) -> (-2767.131, 1348.9582) centre (-2767.0991, 1381.8889) ccw
  arc A293 (-2866.3796, 1403.8421) -> (-2784.1053, 1353.6893) centre (2438.462, 10013.7125) ccw
  arc A294 (-2944.4062, 1453.3364) -> (-2866.3796, 1403.8421) centre (-1013.2028, 4411.586) ccw
  arc A295 (-2995.778, 1489.8358) -> (-2944.4062, 1453.3364) centre (-2506.9157, 2123.4923) ccw
  arc A296 (-3037.5337, 1525.4836) -> (-2995.778, 1489.8358) centre (-2657.1182, 1928.8013) ccw
  arc A297 (-3076.2921, 1565.6566) -> (-3037.5337, 1525.4836) centre (-2631.065, 1956.4224) ccw
  arc A298 (-3109.7189, 1607.7044) -> (-3076.2921, 1565.6566) centre (-2661.4343, 1929.7672) ccw
  arc A299 (-3135.4298, 1648.9509) -> (-3109.7189, 1607.7044) centre (-2808.5529, 1824.0717) ccw
  arc A300 (-3145.0753, 1673.4155) -> (-3135.4298, 1648.9509) centre (-3035.5254, 1702.4737) ccw
  arc A301 (-3151.1847, 1704.6665) -> (-3145.0753, 1673.4155) centre (-2912.5111, 1735.103) ccw
  arc A302 (-3155.1063, 1749.9656) -> (-3151.1847, 1704.6665) centre (-2593.961, 1775.7249) ccw
  arc A303 (-3157.7463, 1823.9509) -> (-3155.1063, 1749.9656) centre (468.79, 1916.3154) ccw
  line L40 (-3157.7463, 1823.9509) -> (-3161.3119, 1963.9509)
  line L41 (-3161.3119, 1963.9509) -> (-3122.9715, 1927.8823)
  arc A304 (-3122.9715, 1927.8823) -> (-3105.0368, 1911.8817) centre (-2811.1062, 2259.3907) ccw
  arc A305 (-3105.0368, 1911.8817) -> (-3082.6506, 1893.5234) centre (-2490.1467, 2638.8564) ccw
  arc A306 (-3082.6506, 1893.5234) -> (-3059.592, 1875.7576) centre (-2486.1369, 2643.9012) ccw
  arc A307 (-3059.592, 1875.7576) -> (-3039.5487, 1861.5653) centre (-2767.5744, 2266.9166) ccw
  arc A308 (3172.093, 1716.3553) -> (3178.3474, 1804.3526) centre (1928.9049, 1848.9355) ccw
  arc A309 (3159.3362, 1658.911) -> (3172.093, 1716.3553) centre (2910.9868, 1744.2012) ccw
  arc A310 (3135.5349, 1611.4892) -> (3159.3362, 1658.911) centre (2972.0304, 1723.2373) ccw
  arc A311 (3094.0019, 1558.7545) -> (3135.5349, 1611.4892) centre (2725.2452, 1891.9039) ccw
  arc A312 (3051.8608, 1518.0929) -> (3094.0019, 1558.7545) centre (2776.8177, 1845.3114) ccw
  arc A313 (2991.5409, 1470.4968) -> (3051.8608, 1518.0929) centre (2252.9148, 2468.598) ccw
  arc A314 (2923.944, 1423.5726) -> (2991.5409, 1470.4968) centre (2183.2354, 2562.755) ccw
  arc A315 (2858.3009, 1384.3286) -> (2923.944, 1423.5726) centre (2370.8302, 2274.2396) ccw
  line L42 (2858.3009, 1384.3286) -> (2791.2328, 1347.5904)
  line L43 (2791.2328, 1347.5904) -> (2788.3009, 1534.0593)
  line L44 (2788.3009, 1534.0593) -> (2785.369, 1720.5281)
  line L45 (2785.369, 1720.5281) -> (2875.369, 1763.9031)
  arc A316 (2875.369, 1763.9031) -> (2951.4796, 1803.139) centre (2183.7754, 3198.9081) ccw
  arc A317 (2951.4796, 1803.139) -> (3023.189, 1845.3617) centre (2266.62, 3048.2829) ccw
  arc A318 (3023.189, 1845.3617) -> (3086.1208, 1887.7557) centre (2379.5862, 2868.6667) ccw
  arc A319 (3086.1208, 1887.7557) -> (3135.2962, 1927.3828) centre (2744.6562, 2361.8231) ccw
  arc A320 (3164.9714, 1949.5013) -> (3135.2962, 1927.3828) centre (3270.2122, 1777.3395) ccw
  arc A321 (3177.4367, 1945.0532) -> (3164.9714, 1949.5013) centre (3169.4079, 1942.2438) ccw
  arc A322 (3181.7451, 1917.6894) -> (3177.4367, 1945.0532) centre (3104.5898, 1919.5624) ccw
  arc A323 (3178.3474, 1804.3526) -> (3181.7451, 1917.6894) centre (-6765.1854, 2159.1688) ccw
  arc A324 (-2409.4291, 1801.5996) -> (-2420.2489, 1810.3134) centre (-2497.2585, 1703.618) ccw
  arc A325 (-2396.9909, 1789.7972) -> (-2409.4291, 1801.5996) centre (-2611.2356, 1576.466) ccw
  arc A326 (-2384.9552, 1777.0089) -> (-2396.9909, 1789.7972) centre (-2617.9113, 1569.8196) ccw
  arc A327 (-2375.3113, 1765.1833) -> (-2384.9552, 1777.0089) centre (-2518.2073, 1658.4958) ccw
  arc A328 (-2363.3504, 1739.1243) -> (-2375.3113, 1765.1833) centre (-2430.1571, 1724.235) ccw
  arc A329 (-2357.6735, 1698.997) -> (-2363.3504, 1739.1243) centre (-2614.7704, 1683.0902) ccw
  arc A330 (-2355.267, 1626.0715) -> (-2357.6735, 1698.997) centre (-3622.0103, 1620.7721) ccw
  arc A331 (-2354.9207, 1435.6164) -> (-2355.267, 1626.0715) centre (-42637.4297, 1457.5953) ccw
  arc A332 (-2355.5061, 1249.212) -> (-2354.9207, 1435.6164) centre (-38285.0681, 1455.2475) ccw
  arc A333 (-2358.0202, 1172.8922) -> (-2355.5061, 1249.212) centre (-3759.5436, 1257.2626) ccw
  arc A334 (-2363.6766, 1129.2945) -> (-2358.0202, 1172.8922) centre (-2676.7557, 1192.0792) ccw
  arc A335 (-2375.1985, 1098.7662) -> (-2363.6766, 1129.2945) centre (-2462.2669, 1149.0658) ccw
  arc A336 (-2426.9729, 1048.4898) -> (-2375.1985, 1098.7662) centre (-2489.7697, 1164.9543) ccw
  arc A337 (-2499.6348, 1030.2743) -> (-2426.9729, 1048.4898) centre (-2499.1399, 1182.3327) ccw
  arc A338 (-2571.5321, 1049.0155) -> (-2499.6348, 1030.2743) centre (-2499.1491, 1179.4185) ccw
  arc A339 (-2621.3584, 1099.5676) -> (-2571.5321, 1049.0155) centre (-2510.4582, 1159.044) ccw
  arc A340 (-2631.5874, 1129.6242) -> (-2621.3584, 1099.5676) centre (-2535.7949, 1145.4559) ccw
  arc A341 (-2636.6921, 1176.1127) -> (-2631.5874, 1129.6242) centre (-2207.4546, 1199.7213) ccw
  arc A342 (-2639.114, 1255.7283) -> (-2636.6921, 1176.1127) centre (-1015.8553, 1265.2616) ccw
  arc A343 (-2639.631, 1431.7915) -> (-2639.114, 1255.7283) centre (27344.0796, 1431.8166) ccw
  arc A344 (-2638.5795, 1638.686) -> (-2639.631, 1431.7915) centre (17716.3772, 1431.7821) ccw
  arc A345 (-2632.9749, 1719.3) -> (-2638.5795, 1638.686) centre (-1956.2478, 1631.7498) ccw
  arc A346 (-2619.129, 1765.5636) -> (-2632.9749, 1719.3) centre (-2484.6388, 1700.1092) ccw
  arc A347 (-2591.7293, 1802.052) -> (-2619.129, 1765.5636) centre (-2511.1479, 1713.0106) ccw
  arc A348 (-2554.3979, 1824.5456) -> (-2591.7293, 1802.052) centre (-2515.6009, 1717.931) ccw
  arc A349 (-2507.8209, 1833.918) -> (-2554.3979, 1824.5456) centre (-2500.1931, 1675.5901) ccw
  arc A350 (-2460.3047, 1829.0798) -> (-2507.8209, 1833.918) centre (-2500.1111, 1673.8877) ccw
  arc A351 (-2420.2489, 1810.3134) -> (-2460.3047, 1829.0798) centre (-2489.8542, 1713.8764) ccw
  arc A352 (2610.5752, 1801.5954) -> (2599.7511, 1810.3134) centre (2522.7668, 1703.653) ccw
  arc A353 (2623.0275, 1789.7787) -> (2610.5752, 1801.5954) centre (2408.2437, 1575.9126) ccw
  arc A354 (2635.0831, 1776.9702) -> (2623.0275, 1789.7787) centre (2401.418, 1569.1163) ccw
  arc A355 (2644.7511, 1765.1204) -> (2635.0831, 1776.9702) centre (2501.1131, 1657.799) ccw
  arc A356 (2656.7516, 1739.3204) -> (2644.7511, 1765.1204) centre (2589.1154, 1723.5512) ccw
  arc A357 (2662.8109, 1699.6609) -> (2656.7516, 1739.3204) centre (2404.2445, 1680.4489) ccw
  arc A358 (2666.0065, 1628.3092) -> (2662.8109, 1699.6609) centre (1451.702, 1609.6717) ccw
  arc A359 (2668.3021, 1448.1596) -> (2666.0065, 1628.3092) centre (-31897.173, 1097.7919) ccw
  arc A360 (2669.5674, 1272.3533) -> (2668.3021, 1448.1596) centre (-27230.0346, 1145.0664) ccw
  arc A361 (2667.8344, 1195.9834) -> (2669.5674, 1272.3533) centre (1251.9717, 1266.3183) ccw
  arc A362 (2662.6197, 1150.2717) -> (2667.8344, 1195.9834) centre (2308.3137, 1213.8434) ccw
  arc A363 (2651.7375, 1114.7157) -> (2662.6197, 1150.2717) centre (2509.0772, 1177.8212) ccw
  arc A364 (2631.9353, 1080.2924) -> (2651.7375, 1114.7157) centre (2479.3821, 1190.9566) ccw
  arc A365 (2607.483, 1055.8878) -> (2631.9353, 1080.2924) centre (2543.5133, 1144.435) ccw
  arc A366 (2576.3755, 1040.1278) -> (2607.483, 1055.8878) centre (2542.0516, 1146.4581) ccw
  arc A367 (2536.6404, 1031.5653) -> (2576.3755, 1040.1278) centre (2513.8394, 1233.8546) ccw
  arc A368 (2498.7701, 1032.0706) -> (2536.6404, 1031.5653) centre (2519.7061, 1181.8051) ccw
  arc A369 (2462.6436, 1042.0121) -> (2498.7701, 1032.0706) centre (2518.8407, 1175.6153) ccw
  arc A370 (2430.772, 1060.6817) -> (2462.6436, 1042.0121) centre (2517.1587, 1171.6167) ccw
  arc A371 (2405.369, 1086.7817) -> (2430.772, 1060.6817) centre (2512.517, 1165.6561) ccw
  arc A372 (2393.7238, 1112.8519) -> (2405.369, 1086.7817) centre (2459.3898, 1126.5479) ccw
  arc A373 (2387.8861, 1155.1921) -> (2393.7238, 1112.8519) centre (2698.8732, 1176.4975) ccw
  arc A374 (2384.7258, 1231.4684) -> (2387.8861, 1155.1921) centre (3798.7808, 1251.8518) ccw
  arc A375 (2382.4609, 1421.1584) -> (2384.7258, 1231.4684) centre (40720.2384, 1784.0612) ccw
  arc A376 (2381.406, 1590.3656) -> (2382.4609, 1421.1584) centre (28558.7262, 1668.9562) ccw
  arc A377 (2382.874, 1677.5923) -> (2381.406, 1590.3656) centre (4581.0643, 1596.9712) ccw
  arc A378 (2386.624, 1730.5384) -> (2382.874, 1677.5923) centre (3161.9536, 1649.0186) ccw
  arc A379 (2394.81, 1757.87) -> (2386.624, 1730.5384) centre (2463.2417, 1722.4826) ccw
  arc A380 (2410.6605, 1781.0527) -> (2394.81, 1757.87) centre (2496.9106, 1705.0717) ccw
  arc A381 (2433.864, 1803.4197) -> (2410.6605, 1781.0527) centre (2559.0601, 1650.3223) ccw
  arc A382 (2460.1721, 1821.5532) -> (2433.864, 1803.4197) centre (2557.3616, 1652.3996) ccw
  arc A383 (2485.369, 1831.9251) -> (2460.1721, 1821.5532) centre (2512.1281, 1731.1263) ccw
  arc A384 (2511.8083, 1834.9909) -> (2485.369, 1831.9251) centre (2509.1565, 1742.3201) ccw
  arc A385 (2544.2906, 1831.4798) -> (2511.8083, 1834.9909) centre (2505.8924, 1628.2527) ccw
  arc A386 (2575.9148, 1822.8731) -> (2544.2906, 1831.4798) centre (2505.7285, 1627.3866) ccw
  arc A387 (2599.7511, 1810.3134) -> (2575.9148, 1822.8731) centre (2543.349, 1732.1694) ccw
  arc A388 (-2005.1347, 1513.0338) -> (-1651.7265, 1458.3197) centre (-857.274, 7758.544) ccw
  arc A389 (-1651.7265, 1458.3197) -> (-1227.043, 1411.9203) centre (-42.9196, 14216.6701) ccw
  arc A390 (-1227.043, 1411.9203) -> (-802.1857, 1379.7439) centre (-46.7944, 14174.9181) ccw
  arc A391 (-802.1857, 1379.7439) -> (-448.5267, 1369.0868) centre (-440.6716, 7503.2617) ccw
  arc A392 (-404.5015, 1368.5678) -> (-448.5267, 1369.0868) centre (-451.2103, -725.9583) ccw
  arc A393 (-359.9619, 1367.1228) -> (-404.5015, 1368.5678) centre (-453.5235, -829.6343) ccw
  arc A394 (-320.7599, 1365.0589) -> (-359.9619, 1367.1228) centre (-443.2041, -587.3167) ccw
  arc A395 (-296.0267, 1362.5917) -> (-320.7599, 1365.0589) centre (-341.9078, 1027.8544) ccw
  line L46 (-296.0267, 1362.5917) -> (-249.631, 1356.2325)
  line L47 (-249.631, 1356.2325) -> (-249.631, 1134.344)
  line L48 (-249.631, 1134.344) -> (-249.631, 912.4556)
  line L49 (-249.631, 912.4556) -> (-362.131, 915.9072)
  arc A396 (-728.9884, 932.2929) -> (-362.131, 915.9072) centre (41.1221, 14059.2879) ccw
  arc A397 (-1074.8528, 958.3398) -> (-728.9884, 932.2929) centre (-116.0078, 11381.0625) ccw
  arc A398 (-1401.2693, 994.1424) -> (-1074.8528, 958.3398) centre (-215.7928, 10296.3864) ccw
  arc A399 (-1709.631, 1039.8703) -> (-1401.2693, 994.1424) centre (-438.29, 8550.4657) ccw
  arc A400 (-1842.1282, 1064.2371) -> (-1709.631, 1039.8703) centre (-917.334, 5720.4984) ccw
  arc A401 (-2002.9151, 1097.4929) -> (-1842.1282, 1064.2371) centre (183.3124, 11262.2501) ccw
  arc A402 (-2155.6865, 1131.1909) -> (-2002.9151, 1097.4929) centre (1130.0123, 15663.8988) ccw
  arc A403 (-2212.3155, 1147.987) -> (-2155.6865, 1131.1909) centre (-2056.9046, 1568.1036) ccw
  arc A404 (-2228.1292, 1165.8661) -> (-2212.3155, 1147.987) centre (-2203.5554, 1171.668) ccw
  arc A405 (-2235.8415, 1214.7987) -> (-2228.1292, 1165.8661) centre (-1908.6823, 1241.2887) ccw
  arc A406 (-2238.2156, 1292.5664) -> (-2235.8415, 1214.7987) centre (-1464.2629, 1277.2739) ccw
  arc A407 (-2234.1063, 1417.1093) -> (-2238.2156, 1292.5664) centre (2471.1796, 1199.5173) ccw
  arc A408 (-2229.8432, 1498.924) -> (-2234.1063, 1417.1093) centre (4763.068, 1093.531) ccw
  arc A409 (-2225.8861, 1534.5982) -> (-2229.8432, 1498.924) centre (-1888.8489, 1479.1561) ccw
  arc A410 (-2220.2869, 1550.937) -> (-2225.8861, 1534.5982) centre (-2174.6567, 1526.171) ccw
  arc A411 (-2211.5622, 1554.157) -> (-2220.2869, 1550.937) centre (-2214.0887, 1547.5729) ccw
  arc A412 (-2211.5622, 1554.157) -> (-2199.7051, 1550.7014) centre (-2184.8204, 1623.8449) ccw
  arc A413 (-2199.7051, 1550.7014) -> (-2144.3555, 1539.5565) centre (533.0518, 14979.4812) ccw
  arc A414 (-2144.3555, 1539.5565) -> (-2079.2863, 1526.8931) centre (-681.907, 8880.656) ccw
  arc A415 (-2079.2863, 1526.8931) -> (-2005.1347, 1513.0338) centre (258.4599, 13829.3081) ccw
  arc A416 (126.5668, 1502.7677) -> (87.3835, 1539.3558) centre (18.3733, 1426.1754) ccw
  arc A417 (146.3037, 1454.9003) -> (126.5668, 1502.7677) centre (31.8331, 1435.7039) ccw
  arc A418 (153.9965, 1368.6196) -> (146.3037, 1454.9003) centre (-407.3525, 1362.0533) ccw
  arc A419 (155.369, 1133.9509) -> (153.9965, 1368.6196) centre (-19909.1522, 1133.9384) ccw
  arc A420 (154.8613, 945.1025) -> (155.369, 1133.9509) centre (-34972.8795, 1133.9611) ccw
  arc A421 (152.4711, 860.2025) -> (154.8613, 945.1025) centre (-1710.3871, 955.1312) ccw
  arc A422 (147.503, 811.0309) -> (152.4711, 860.2025) centre (-343.4967, 885.476) ccw
  arc A423 (137.3835, 781.0087) -> (147.503, 811.0309) centre (57.3627, 824.6978) ccw
  arc A424 (83.8015, 727.9305) -> (137.3835, 781.0087) centre (21.7802, 844.1247) ccw
  arc A425 (6.5664, 709.0683) -> (83.8015, 727.9305) centre (8.3671, 869.2539) ccw
  arc A426 (-68.0852, 729.8331) -> (6.5664, 709.0683) centre (8.2603, 859.7311) ccw
  arc A427 (-115.2328, 783.8487) -> (-68.0852, 729.8331) centre (-10.6578, 827.5429) ccw
  arc A428 (-122.7453, 814.128) -> (-115.2328, 783.8487) centre (-20.538, 823.4148) ccw
  arc A429 (-126.7449, 874.806) -> (-122.7453, 814.128) centre (1098.6095, 925.1039) ccw
  arc A430 (-129.0352, 969.7228) -> (-126.7449, 874.806) centre (2680.1003, 990.0217) ccw
  arc A431 (-129.631, 1134.6185) -> (-129.0352, 969.7228) centre (22684.0456, 1134.5998) ccw
  arc A432 (-128.1958, 1364.9408) -> (-129.631, 1134.6185) centre (18349.9179, 1134.6283) ccw
  arc A433 (-120.5666, 1454.7503) -> (-128.1958, 1364.9408) centre (495.7759, 1357.1639) ccw
  arc A434 (-101.8129, 1504.3665) -> (-120.5666, 1454.7503) centre (8.5169, 1434.3122) ccw
  arc A435 (-65.4314, 1540.0942) -> (-101.8129, 1504.3665) centre (-6.892, 1444.0961) ccw
  arc A436 (-31.0953, 1553.9676) -> (-65.4314, 1540.0942) centre (-6.2425, 1443.031) ccw
  arc A437 (10.7306, 1558.493) -> (-31.0953, 1553.9676) centre (9.8259, 1371.3062) ccw
  arc A438 (52.6771, 1553.559) -> (10.7306, 1558.493) centre (9.8196, 1369.9769) ccw
  arc A439 (87.3835, 1539.3558) -> (52.6771, 1553.559) centre (25.7719, 1438.3095) ccw
  arc A440 (2259.0761, 1226.977) -> (2259.4801, 1358.5344) centre (-19166.9629, 1358.5471) ccw
  arc A441 (2256.5961, 1182.9366) -> (2259.0761, 1226.977) centre (1818.78, 1229.6812) ccw
  arc A442 (2250.1702, 1161.3021) -> (2256.5961, 1182.9366) centre (2194.7222, 1189.5428) ccw
  arc A443 (2237.1765, 1149.6382) -> (2250.1702, 1161.3021) centre (2228.5566, 1172.3103) ccw
  arc A444 (2179.6212, 1132.2035) -> (2237.1765, 1149.6382) centre (2082.6059, 1556.1887) ccw
  arc A445 (2028.0515, 1098.4497) -> (2179.6212, 1132.2035) centre (-792.9628, 14123.2595) ccw
  arc A446 (1866.8261, 1064.9729) -> (2028.0515, 1098.4497) centre (-7.4886, 10496.7099) ccw
  arc A447 (1730.369, 1039.8703) -> (1866.8261, 1064.9729) centre (917.4772, 5842.166) ccw
  arc A448 (1419.6925, 993.8376) -> (1730.369, 1039.8703) centre (456.9829, 8562.6077) ccw
  arc A449 (1089.9832, 957.7448) -> (1419.6925, 993.8376) centre (222.512, 10406.1137) ccw
  arc A450 (743.6158, 931.772) -> (1089.9832, 957.7448) centre (139.5994, 11309.3507) ccw
  arc A451 (382.869, 916.1549) -> (743.6158, 931.772) centre (38.2892, 13050.0525) ccw
  line L50 (382.869, 916.1549) -> (280.369, 913.244)
  line L51 (280.369, 913.244) -> (280.369, 1135.2443)
  line L52 (280.369, 1135.2443) -> (280.369, 1357.2445)
  line L53 (280.369, 1357.2445) -> (352.869, 1362.7749)
  arc A452 (393.159, 1365.2702) -> (352.869, 1362.7749) centre (460.3793, -46.6215) ccw
  arc A453 (462.8221, 1368.3708) -> (393.159, 1365.2702) centre (929.0511, -9890.9224) ccw
  arc A454 (543.4822, 1371.45) -> (462.8221, 1368.3708) centre (980.4076, -11131.6163) ccw
  arc A455 (625.369, 1374.0585) -> (543.4822, 1371.45) centre (1007.059, -11894.6817) ccw
  arc A456 (625.369, 1374.0585) -> (987.2456, 1390.9224) centre (332.9072, 11541.0526) ccw
  arc A457 (987.2456, 1390.9224) -> (1347.9367, 1420.6521) centre (335.4512, 11501.5848) ccw
  arc A458 (1347.9367, 1420.6521) -> (1697.3081, 1462.2224) centre (388.7771, 10970.681) ccw
  arc A459 (1697.3081, 1462.2224) -> (2025.1358, 1514.6454) centre (659.5528, 9003.0755) ccw
  arc A460 (2025.1358, 1514.6454) -> (2098.769, 1528.2319) centre (-1197.7418, 19187.7414) ccw
  arc A461 (2098.769, 1528.2319) -> (2162.4255, 1540.3261) centre (245.5849, 11455.7731) ccw
  arc A462 (2162.4255, 1540.3261) -> (2217.5398, 1551.039) centre (-3071.7301, 28615.6019) ccw
  arc A463 (2217.5398, 1551.039) -> (2225.369, 1553.3542) centre (2209.244, 1593.4877) ccw
  arc A464 (2243.9277, 1551.9732) -> (2225.369, 1553.3542) centre (2233.2417, 1533.7596) ccw
  arc A465 (2254.7674, 1536.3569) -> (2243.9277, 1551.9732) centre (2232.4756, 1532.4538) ccw
  arc A466 (2258.8241, 1492.182) -> (2254.7674, 1536.3569) centre (1987.2428, 1489.5158) ccw
  arc A467 (2259.4801, 1358.5344) -> (2258.8241, 1492.182) centre (-11356.0379, 1358.53) ccw
  arc A468 (-2964.8997, 1324.4876) -> (-2934.0089, 1305.0613) centre (-2458.0456, 2096.1884) ccw
  arc A469 (-2934.0089, 1305.0613) -> (-2896.9573, 1283.3808) centre (-2026.3893, 2813.6696) ccw
  arc A470 (-2896.9573, 1283.3808) -> (-2859.7972, 1262.8378) centre (-2038.135, 2793.0177) ccw
  arc A471 (-2859.7972, 1262.8378) -> (-2828.6701, 1246.9876) centre (-2480.7397, 1968.7533) ccw
  line L54 (-2828.6701, 1246.9876) -> (-2760.1372, 1213.9509)
  line L55 (-2760.1372, 1213.9509) -> (-2759.7864, 1163.9509)
  arc A472 (-2759.7864, 1163.9509) -> (-2747.0054, 1092.6387) centre (-2546.0874, 1165.4499) ccw
  arc A473 (-2747.0054, 1092.6387) -> (-2710.4741, 1022.0475) centre (-2458.5163, 1197.1852) ccw
  arc A474 (-2710.4741, 1022.0475) -> (-2657.326, 963.6152) centre (-2461.5352, 1195.087) ccw
  arc A475 (-2657.326, 963.6152) -> (-2595.7776, 928.0039) centre (-2527.3238, 1117.3094) ccw
  line L56 (-2595.7776, 928.0039) -> (-2559.631, 914.9332)
  line L57 (-2559.631, 914.9332) -> (-2559.631, -710.6165)
  line L58 (-2559.631, -710.6165) -> (-2559.631, -2336.1661)
  line L59 (-2559.631, -2336.1661) -> (-2611.6897, -2360.0485)
  line L60 (-2611.6897, -2360.0485) -> (-2663.7483, -2383.9308)
  line L61 (-2663.7483, -2383.9308) -> (-2713.4763, -2329.9899)
  arc A476 (-2772.0631, -2261.8128) -> (-2713.4763, -2329.9899) centre (-1766.3177, -1456.805) ccw
  arc A477 (-2828.8817, -2186.2844) -> (-2772.0631, -2261.8128) centre (-1543.3745, -1278.3571) ccw
  arc A478 (-2880.3127, -2108.5599) -> (-2828.8817, -2186.2844) centre (-1575.1805, -1300.8213) ccw
  arc A479 (-2922.6665, -2033.8042) -> (-2880.3127, -2108.5599) centre (-1936.764, -1524.6046) ccw
  arc A480 (-2922.6665, -2033.8042) -> (-2953.0118, -1978.0113) centre (-4241.3846, -2714.8959) ccw
  arc A481 (-2953.0118, -1978.0113) -> (-2973.6055, -1949.8578) centre (-3088.4648, -2055.4838) ccw
  arc A482 (-2973.6055, -1949.8578) -> (-2993.2412, -1935.9575) centre (-3015.8349, -1988.6925) ccw
  arc A483 (-2993.2412, -1935.9575) -> (-3017.1615, -1931.0491) centre (-3017.1615, -1991.7888) ccw
  arc A484 (-3017.1615, -1931.0491) -> (-3034.6762, -1935.6138) centre (-3017.1615, -1966.9333) ccw
  arc A485 (-3034.6762, -1935.6138) -> (-3052.1608, -1949.047) centre (-2997.4877, -2002.1135) ccw
  arc A486 (-3052.1608, -1949.047) -> (-3065.192, -1967.0592) centre (-2996.6498, -2002.9269) ccw
  arc A487 (-3065.192, -1967.0592) -> (-3069.6231, -1985.0989) centre (-3030.7466, -1985.0843) ccw
  arc A488 (-3069.6231, -1985.0989) -> (-3054.6183, -2045.8273) centre (-2939.0308, -1985.0498) ccw
  arc A489 (-3054.6183, -2045.8273) -> (-2990.6524, -2157.8219) centre (-1416.5898, -1184.5293) ccw